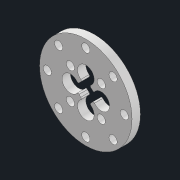
# Autodesk Inventor part: s_base5
Saved by Autodesk Inventor 2022 (Build 260153000, 153)
## iProperties
Created: 2021-08-27
Part Number: s_base5
Material: 一般
Document SubType Name: Modeling
Designer: Yuta Kage
Density: 1 g/cm^3
Appearance: 既定
Author: Yuta Kage
Autodesk Inventor part; units mm, degrees
ref_plane "YZ Plane" through (0, 0, 0) normal (1, 0, 0) x (0, 1, 0)
ref_plane "XZ Plane" through (0, 0, 0) normal (0, 1, 0) x (-1, 0, 0)
ref_plane "XY Plane" through (0, 0, 0) normal (0, 0, 1) x (1, 0, 0)
sketch "スケッチ1" plane through (0, 0, 0) normal (0, 0, 1) x (1, 0, 0)
  circle A0 centre (0, 0) radius 18
  dimension "d0" = 36
  constraints: 1 centre point, 1 coincident
  measures "d0" diameter of A0
extrude "押し出し1" add sketch "スケッチ1" along normal blind 3.25
sketch "スケッチ2" plane through (0, 0, 3.25) normal (0, 0, 1) x (1, 0, 0)
  circle A0 centre (0, 0) radius 6
  point P0 (0, 6)
  point P1 (-6, 0)
  point P2 (0, -6)
  point P3 (6, 0)
  dimension "d3" = 12
  dimension "d6" = 360
  constraints: 1 coincident, 1 vertical alignment, 7 other
hole "穴1" at (0, 6, 3.25) at (-6, 0, 3.25) at (0, -6, 3.25) at (6, 0, 3.25) direction (0, 0, -1) diameter 3.2 end through all counterbore diameter 6.5 counterbore depth 4 clearance for "Socket Head Cap Screw" size "M3" standard "Ansi Metric M Profile"
sketch "スケッチ3" plane through (0, 0, 0) normal (0, 0, -1) x (-1, 0, 0)
  circle A0 centre (0, 0) radius 8.5
  point P0 (-6.0104, 6.0104)
  point P1 (-6.0104, -6.0104)
  point P2 (6.0104, -6.0104)
  point P3 (6.0104, 6.0104)
  dimension "d15" = 17
  dimension "d18" = 360
  constraints: 1 coincident, 1 horizontal alignment, 8 other
hole "穴2" at (6.0104, 6.0104, 0) at (6.0104, -6.0104, 0) at (-6.0104, -6.0104, 0) at (-6.0104, 6.0104, 0) direction (0, 0, 1) diameter 3.2 end through all clearance for "Socket Head Cap Screw" size "M3" standard "Ansi Metric M Profile"
sketch "スケッチ4" plane through (0, 0, 0) normal (0, 0, -1) x (-1, 0, 0)
  circle A0 centre (0, 0) radius 3.25
  dimension "d27" = 6.5
  constraints: 1 centre point, 1 coincident
  measures "d27" diameter of A0
extrude "押し出し2" cut sketch "スケッチ4" against normal blind 8
fillet "フィレット1" radius 0.5 8 edges at (-1.25, -3, 1.625) (1.25, -3, 1.625) (3, -1.25, 1.625) (3, 1.25, 1.625) (1.25, 3, 1.625) (-1.25, 3, 1.625) (-3, 1.25, 1.625) (-3, -1.25, 1.625)
sketch "スケッチ5" plane through (0, 0, 3.25) normal (0, 0, 1) x (1, 0, 0)
  circle A0 centre (0, 0) radius 15
  point P0 (0, -15)
  point P1 (10.6066, -10.6066)
  point P2 (15, 0)
  point P3 (10.6066, 10.6066)
  point P4 (0, 15)
  point P5 (-10.6066, 10.6066)
  point P6 (-15, 0)
  point P7 (-10.6066, -10.6066)
  dimension "d31" = 30
  dimension "d34" = 360
  constraints: 1 coincident, 1 vertical alignment, 11 other
hole "穴3" at (0, -15, 3.25) at (10.6066, -10.6066, 3.25) at (15, 0, 3.25) at (10.6066, 10.6066, 3.25) at (0, 15, 3.25) at (-10.6066, 10.6066, 3.25) at (-15, 0, 3.25) at (-10.6066, -10.6066, 3.25) direction (0, 0, -1) diameter 3.2 end through all clearance for "Socket Head Cap Screw" size "M3" standard "Ansi Metric M Profile"
